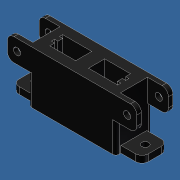
# Autodesk Inventor part: TB-22PP
Saved by Autodesk Inventor 2016 (Build 200138000, 138)
## iProperties
Created: 2011-02-27
Part Number: TB-22PP
Material: ABS Plastic
Document SubType Name: Modeling
Designer: Nishioka
Mass: 5.23483 g
Surface Area: 28.2374 cm^2
Volume: 4.93852 cm^3
Density: 1.06 g/cm^3
Appearance: 光沢 - 黒
Author: Nishioka
Autodesk Inventor part; units mm, degrees
ref_plane "YZ Plane" through (0, 0, 0) normal (1, 0, 0) x (0, 1, 0)
ref_plane "XZ Plane" through (0, 0, 0) normal (0, 1, 0) x (-1, 0, 0)
ref_plane "XY Plane" through (0, 0, 0) normal (0, 0, 1) x (1, 0, 0)
sketch "スケッチ1" plane through (0, 0, 0) normal (0, 0, 1) x (1, 0, 0)
  line L0 (-39.4908, -6.839) -> (0.6092, -6.839)
  line L1 (0.6092, -6.839) -> (0.6092, -18.039)
  line L2 (0.6092, -18.039) -> (-39.4908, -18.039)
  line L3 (-39.4908, -18.039) -> (-39.4908, -6.839)
  point P0 (0, 0)
  dimension "d0" = 40.1
  dimension "d1" = 11.2
  constraints: 8 end point, 2 parallel, 1 horizontal, 1 perpendicular
  measures "d0" distance of L1.end L2.end
  measures "d1" distance of L0.end L1.end
extrude "押し出し1" add sketch "スケッチ1" along normal blind 16.3
sketch "スケッチ2" plane through (0.6092, -18.039, 0) normal (1, 0, 0) x (0, 0, -1)
  line L0 (-16.3, 11.2) -> (-16.3, 0) projected
  line L1 (0, 0) -> (-16.3, 0) projected
  line L2 (0, 11.2) -> (0, 0) projected
  line L3 (0, 11.2) -> (-16.3, 11.2) projected
  line L4 (-16.3, 0) -> (-9.3, 0)
  line L5 (-9.3, 0) -> (-9.3, 1.4)
  line L6 (-9.3, 1.4) -> (-16.3, 1.4)
  line L7 (-16.3, 1.4) -> (-16.3, 0)
  line L8 (-16.3, 11.2) -> (-9.3, 11.2)
  line L9 (-9.3, 11.2) -> (-9.3, 9.8)
  line L10 (-9.3, 9.8) -> (-16.3, 9.8)
  line L11 (-16.3, 9.8) -> (-16.3, 11.2)
  line L12 (0, 1.6) -> (-2.1, 1.6)
  line L13 (-2.1, 1.6) -> (-2.1, 9.6)
  line L14 (-2.1, 9.6) -> (0, 9.6)
  line L15 (0, 9.6) -> (0, 1.6)
  point P0 (0, 18.039)
  dimension "d4" = 8
  dimension "d5" = 2.1
  dimension "d6" = 7
  dimension "d7" = 7
  dimension "d8" = 8.4
  constraints: 24 end point, 6 parallel, 3 horizontal, 3 perpendicular, 1 point on line
  measures "d4" distance between parallel lines of L12 L14
  measures "d5" distance between parallel lines of L13 L2
  measures "d6" distance of L9.end L10.end
  measures "d7" distance of L5.end L6.end
  measures "d8" distance between parallel lines of L10 L6
extrude "押し出し2" cut sketch "スケッチ2" against normal blind 6.5 contours L10 L9 L3 L2 L14 L13 L12 L1 L5 L6 L0
sketch "スケッチ3" plane through (-39.4908, -18.039, 0) normal (-1, 0, 0) x (0, 0, 1)
  line L0 (16.3, 0) -> (16.3, 11.2) projected
  line L1 (0, 11.2) -> (16.3, 11.2) projected
  line L2 (0, 0) -> (0, 11.2) projected
  line L3 (0, 0) -> (16.3, 0) projected
  line L4 (16.3, 11.2) -> (9.3, 11.2)
  line L5 (9.3, 11.2) -> (9.3, 9.8)
  line L6 (9.3, 9.8) -> (16.3, 9.8)
  line L7 (16.3, 9.8) -> (16.3, 11.2)
  line L8 (16.3, 0) -> (9.3, 0)
  line L9 (9.3, 0) -> (9.3, 1.4)
  line L10 (9.3, 1.4) -> (16.3, 1.4)
  line L11 (16.3, 1.4) -> (16.3, 0)
  line L12 (0, 9.6) -> (2.1, 9.6)
  line L13 (2.1, 9.6) -> (2.1, 1.6)
  line L14 (2.1, 1.6) -> (0, 1.6)
  line L15 (0, 1.6) -> (0, 9.6)
  line L16 (2.1, 5.6) -> (16.3, 5.6)
  point P0 (0, 18.039)
  dimension "d12" = 7
  dimension "d13" = 7
  dimension "d14" = 8
  dimension "d15" = 2.1
  dimension "d16" = 8.4
  dimension "d17" = 4.2
  constraints: 26 end point, 6 parallel, 4 perpendicular, 3 horizontal, 2 midpoint, 1 point on line
  measures "d12" distance of L9.end L10.end
  measures "d13" distance of L5.end L6.end
  measures "d14" distance of L12.end L13.end
  measures "d15" distance between parallel lines of L13 L15
  measures "d16" distance between parallel lines of L10 L6
  measures "d17" distance between parallel lines of L16 L10
extrude "押し出し3" cut sketch "スケッチ3" against normal blind 6.5 contours L10 L9 L3 L2 L14 L13 L16 L0 | L16 L13 L12 L2 L1 L5 L6 L0
sketch "スケッチ4" plane through (0, 0, 0) normal (0, 0, -1) x (-1, 0, 0)
  line L0 (5.8908, -18.039) -> (32.9908, -18.039) projected
  line L1 (39.4908, -8.439) -> (32.9908, -8.439) projected
  line L2 (36.4908, -12.439) -> (2.3908, -12.439)
  line L3 (19.4408, -12.439) -> (19.4408, -18.039)
  point P0 (0, 0)
  dimension "d20" = 34.1
  dimension "d21" = 5.6
  constraints: 4 end point, 2 midpoint, 1 parallel, 1 perpendicular
  measures "d20" distance of L2.start L2.end
  measures "d21" distance between parallel lines of L0 L2
hole "穴1" at (-36.4908, -12.439, 0) at (-2.3908, -12.439, 0) direction (0, 0, 1) diameter 2.2 end through all
sketch "スケッチ5" plane through (-39.4908, -18.039, 16.3) normal (0, -1, 0) x (1, 0, 0)
  line L0 (33.6, -16.3) -> (6.5, -16.3) projected
  line L1 (40.1, -7) -> (40.1, 0) projected
  line L2 (40.1, 0) -> (0, 0) projected
  line L3 (3, -3.5) -> (37.1, -3.5)
  line L4 (20.05, -3.5) -> (20.05, 0)
  point P0 (39.4908, -16.3)
  dimension "d29" = 34.1
  dimension "d30" = 12.8
  constraints: 4 end point, 2 midpoint, 2 perpendicular
  measures "d29" distance of L3.start L3.end
  measures "d30" distance between parallel lines of L0 L3
hole "穴2" at (-36.4908, -18.039, 12.8) at (-2.3908, -18.039, 12.8) direction (0, 1, 0) diameter 2.2 end through all
fillet "フィレット1" radius 2 12 edges at (0.6092, -17.339, 16.3) (0.6092, -17.339, 9.3) (0.6092, -7.539, 16.3) (0.6092, -7.539, 9.3) (-39.4908, -7.539, 16.3) (-39.4908, -17.339, 16.3) (-39.4908, -17.339, 9.3) (-39.4908, -7.539, 9.3) (0.6092, -16.439, 1.05) (0.6092, -8.439, 1.05) (-39.4908, -16.439, 1.05) (-39.4908, -8.439, 1.05)
fillet "フィレット2" radius 1 4 edges at (-32.9908, -18.039, 4.65) (-5.8908, -18.039, 4.65) (-5.8908, -6.839, 4.65) (-32.9908, -6.839, 4.65)
sketch "スケッチ6" plane through (0, 0, 16.3) normal (0, 0, 1) x (1, 0, 0)
  line L0 (-29.4408, -9.939) -> (-21.4408, -9.939)
  line L1 (-21.4408, -9.939) -> (-21.4408, -14.939)
  line L2 (-21.4408, -14.939) -> (-29.4408, -14.939)
  line L3 (-9.4408, -9.939) -> (-17.4408, -9.939)
  line L4 (-17.4408, -9.939) -> (-17.4408, -14.939)
  line L5 (-17.4408, -14.939) -> (-9.4408, -14.939)
  line L6 (-29.4408, -9.939) -> (-30.4408, -9.939)
  line L7 (-30.4408, -9.939) -> (-30.4408, -10.939)
  line L8 (-30.4408, -10.939) -> (-29.4408, -10.939)
  line L9 (-29.4408, -12.439) -> (-30.4408, -12.439)
  line L10 (-30.4408, -12.439) -> (-30.4408, -13.439)
  line L11 (-30.4408, -13.439) -> (-29.4408, -13.439)
  line L12 (-9.4408, -14.939) -> (-8.4408, -14.939)
  line L13 (-8.4408, -14.939) -> (-8.4408, -13.939)
  line L14 (-8.4408, -13.939) -> (-9.4408, -13.939)
  line L15 (-9.4408, -12.439) -> (-8.4408, -12.439)
  line L16 (-8.4408, -12.439) -> (-8.4408, -11.439)
  line L17 (-8.4408, -11.439) -> (-9.4408, -11.439)
  line L18 (-29.4408, -14.939) -> (-29.4408, -13.439)
  line L19 (-29.4408, -12.439) -> (-29.4408, -10.939)
  line L20 (-9.4408, -13.939) -> (-9.4408, -12.439)
  line L21 (-9.4408, -11.439) -> (-9.4408, -9.939)
  point P0 (0, 0)
  dimension "d41" = 5
  dimension "d43" = 1
  dimension "d46" = 1
  dimension "d47" = 1
  dimension "d50" = 1
  constraints: 44 end point, 7 parallel, 5 horizontal, 5 perpendicular
  measures "d41" distance between parallel lines of L0 L2
  measures "d43" distance between parallel lines of L6 L8
  measures "d46" distance between parallel lines of L9 L11
  measures "d47" distance between parallel lines of L17 L15
  measures "d50" distance between parallel lines of L14 L12
extrude "押し出し4" cut sketch "スケッチ6" against normal blind 5
